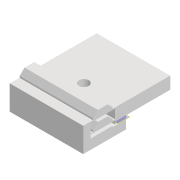
# Autodesk Inventor part: 11_SSOCT_sample_linearflexure_v0
Saved by Autodesk Inventor 2022 (Build 260153000, 153)
## iProperties
Created: 2023-01-12
Part Number: 11_SSOCT_sample_linearflexure_v0
Material: Generisch
Document SubType Name: Modeling
Designer: diederichbenedict
Density: 1 g/cm^3
Appearance: Vorgabe
Author: diederichbenedict
Autodesk Inventor part; units mm, degrees
ref_plane "YZ Plane" through (0, 0, 0) normal (1, 0, 0) x (0, 1, 0)
ref_plane "XZ Plane" through (0, 0, 0) normal (0, 1, 0) x (-1, 0, 0)
ref_plane "XY Plane" through (0, 0, 0) normal (0, 0, 1) x (1, 0, 0)
sketch "Skizze1" plane through (0, 0, 0) normal (1, 0, 0) x (0, 1, 0)
  line L0 (0, 0) -> (4, 0)
  line L1 (4, 0) -> (4, 12)
  line L2 (4, 12) -> (0, 12)
  line L3 (0, 12) -> (0, 0)
  line L4 (10, 9) -> (4, 9)
  line L5 (4, 9) -> (4, 12)
  line L6 (12.6, 8) -> (9.6, 8)
  line L7 (9.6, 8) -> (9.6, 0)
  line L8 (9.6, 0) -> (12.6, 0)
  line L9 (12.6, 0) -> (12.6, 8)
  line L10 (8.4, 8) -> (5.4, 8)
  line L11 (5.4, 8) -> (5.4, 0)
  line L12 (5.4, 0) -> (8.4, 0)
  line L13 (8.4, 0) -> (8.4, 8)
  line L14 (9.6, 8) -> (10, 8)
  line L15 (10, 8) -> (10, 9)
  line L16 (10, 9) -> (9.6, 9)
  line L17 (9.6, 9) -> (9.6, 8)
  line L18 (5.4, 8) -> (5.8, 8)
  line L19 (5.8, 8) -> (5.8, 9)
  line L20 (5.8, 9) -> (5.4, 9)
  line L21 (5.4, 9) -> (5.4, 8)
  line L22 (9.6, 0) -> (10, 0)
  line L23 (10, 0) -> (10, -1)
  line L24 (10, -1) -> (9.6, -1)
  line L25 (9.6, -1) -> (9.6, 0)
  line L26 (5.4, 0) -> (5.8, 0)
  line L27 (5.8, 0) -> (5.8, -1)
  line L28 (5.8, -1) -> (5.4, -1)
  line L29 (5.4, -1) -> (5.4, 0)
  line L30 (10, -1) -> (4, -1)
  line L31 (4, -1) -> (4, -5.5)
  line L32 (4, -5.5) -> (10, -5.5)
  line L33 (10, -5.5) -> (10, -1)
  line L34 (4, 9) -> (10, 9)
  line L35 (10, 9) -> (10, 12)
  line L36 (10, 12) -> (4, 12)
  line L37 (4, 12) -> (4, 9)
  line L38 (0, 0) -> (3.5, 0)
  line L39 (3.5, 0) -> (3.5, -5.5)
  line L40 (3.5, -5.5) -> (0, -5.5)
  line L41 (0, -5.5) -> (0, 0)
  point P0 (4, 9)
  point P1 (5.4, 9)
  point P2 (5.4, -1)
  point P3 (10, 0)
  point P4 (5.8, -1)
  point P5 (5.8, 0)
  point P6 (4, 10)
  dimension "d0" = 4
  dimension "d1" = 12
  dimension "d4" = 3
  dimension "d5" = 8
  dimension "d6" = 3
  dimension "d7" = 0.4
  dimension "d8" = 0.4
  dimension "d9" = 0.4
  dimension "d10" = 1
  dimension "d11" = 0.4
  dimension "d12" = 1
  dimension "d13" = 4.5
  dimension "d25" = 1
  dimension "d26" = 6
  dimension "d27" = 3
  dimension "d28" = 1.2
  dimension "d29" = 6
  dimension "d38" = 3.5
  constraints: 84 end point, 20 parallel, 10 perpendicular, 9 horizontal, 3 point on line
  measures "d0" distance of L2.end L1.end
  measures "d1" distance of L1.end L0.end
  measures "d4" distance of L8.end L7.end
  measures "d5" distance of L7.end L6.end
  measures "d6" distance of L12.end L11.end
  measures "d7" distance of L4.start L16.end
  measures "d8" distance of L20.end L19.end
  measures "d9" distance of L23.end L24.end
  measures "d10" distance of L22.end L23.end
  measures "d11" distance between parallel lines of L27 L29
  measures "d12" distance of L11.end L28.end
  measures "d13" distance of L31.end L30.end
  measures "d25" distance between parallel lines of L6 L4
  measures "d26" distance between parallel lines of L35 L1
  measures "d27" distance between parallel lines of L36 L4
  measures "d28" distance between parallel lines of L13 L7
  measures "d29" distance between parallel lines of L31 L33
  measures "d38" distance of L39.end L40.end
extrude "Extrusion1" add sketch "Skizze1" along normal blind 30 contours L3 L2 L1 L0 | L0 L39 L40 L41 | L36 L35 L4 L1 | L4 L19 L10 L21 | L15 L6 L17 L4 | L10 L13 L12 L11 | L6 L9 L8 L7 | L12 L27 L28 L29 | L28 L30 L24 L33 L32 L31 | L8 L23 L24 L25
chamfer "Fase1" distance 2 angle 45 4 edges at (15, 12.6, 0) (15, 12.6, 8) (15, 8.4, 8) (15, 8.4, 0)
sketch "Skizze2" plane through (0, 0, 0) normal (0, -1, 0) x (1, 0, 0)
  circle A0 centre (22, 4) radius 4
  circle A1 centre (8, 4) radius 4
  line L0 (0, 12) -> (30, 12) projected
  point P0 (0, 0)
  dimension "d19" = 8
  dimension "d20" = 8
  dimension "d39" = 8
  dimension "d40" = 0
  constraints: 2 centre point
  measures "d19" diameter of A0
  measures "d20" diameter of A1
  measures "d39" distance from line of L0 A0.centre
  measures "d40" vertical distance of A0.centre A1.centre
extrude "Extrusion2" cut sketch "Skizze2" against normal blind 3
sketch "Skizze3" plane through (0, 10, 0) normal (0, 1, 0) x (1, 0, 0)
  line L0 (0, 5.5) -> (0, 0) projected
  line L1 (0, 0) -> (30, 0) projected
  line L2 (30, 5.5) -> (30, 0) projected
  line L3 (0, 5.5) -> (30, 5.5) projected
  line L4 (0, 1) -> (30, 1) projected
  circle A0 centre (15, 3.25) radius 2.25
  line L5 (30, 5.5) -> (30, 0) projected
  point P0 (0, 0)
  dimension "d30" = 4.5
  dimension "d41" = 15
  constraints: 1 centre point, 1 tangent
  measures "d30" diameter of A0
  measures "d41" distance from line of L5 A0.centre
hole "Bohrung1" at (15, 10, -3.25) direction (0, -1, 0) diameter 3.4 depth 6 tip angle 118 counterbore diameter 4 counterbore depth 6
ref_plane "Arbeitsebene1" through (0, 5, -5.5) normal (0, -1, 0) x (1, 0, 0)
sketch "Skizze4" plane through (0, 5, -5.5) normal (0, -1, 0) x (1, 0, 0)
  circle A0 centre (8, 9.5) radius 4 projected
  circle A1 centre (22, 9.5) radius 4 projected
  line L0 (0, 17.5) -> (0, 0) projected
  line L1 (0, 0) -> (30, 0) projected
  line L2 (30, 17.5) -> (30, 0) projected
  line L3 (0, 17.5) -> (30, 17.5) projected
  line L4 (0, -18) -> (30, -18)
  line L5 (30, -18) -> (30, 0)
  line L6 (30, 0) -> (0, 0)
  line L7 (0, 0) -> (0, -18)
  line L8 (0, -18) -> (30, 0) construction
  line L9 (30, -18) -> (0, 0) construction
  line L10 (0, 0) -> (30, 0) projected
  point P0 (0, 5.5)
  point P1 (15, -9)
  point P2 (27, 0)
  point P3 (3, 0)
  dimension "d44" = 18
  constraints: 12 end point, 3 point on line, 2 midpoint, 2 parallel, 1 horizontal, 1 perpendicular
  measures "d44" distance of L5.end L4.end
extrude "Extrusion3" add sketch "Skizze4" against normal up to surface (5 mm away) contours L1 L5 L4 L7
equation "\"d8\" = d7"
equation "\"d9\" = d7"
equation "\"d11\" = d7"
